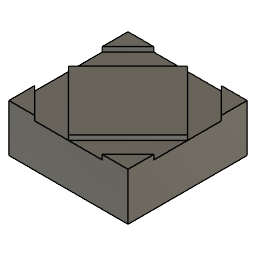
Tugas CNC Milling (Autodesk Fusion 360 design; units mm, degrees)
part number: 2026-05-23-22-12-12-129
Autodesk Fusion 360 part; units mm, degrees
sketch "Sketch1" plane through (0, 0, 0) normal (0, 0, 1) x (1, 0, 0)
  line L0 (0, 0) -> (50, 0)
  line L1 (50, 0) -> (50, 50)
  line L2 (50, 50) -> (0, 50)
  line L3 (0, 50) -> (0, 0)
  dimension "d1" = 50
  dimension "d2" = 50
  constraint horizontal L0
  constraint vertical L1
  constraint horizontal L2
  constraint vertical L3
  constraint coincident L0.start L3.end
  measures "d1" distance of L0.end L1.end
  measures "d2" distance of L1.end L2.end
extrude "Extrude1" add sketch "Sketch1" along normal blind 20
sketch "Sketch2" plane through (0, 0, 20) normal (0, 0, 1) x (-1, 0, 0)
  line L0 (0, -50) -> (0, 0)
  line L1 (0, 0) -> (-50, 0)
  line L2 (-50, 0) -> (-50, -50)
  line L3 (-50, -50) -> (0, -50)
  line L4 (-25, 0) -> (0, -25)
  line L5 (0, -25) -> (-25, -50)
  line L6 (-25, -50) -> (-50, -25)
  line L7 (-50, -25) -> (-25, 0)
  line L8 (0, -10.8579) -> (-10.8579, 0)
  line L9 (-39.1421, 0) -> (-50, -10.8579)
  line L10 (-50, -39.1421) -> (-39.1421, -50)
  line L11 (-10.8579, -50) -> (0, -39.1421)
  line L12 (0, -10.8579) -> (0, -39.1421)
  line L13 (-10.8579, -50) -> (-39.1421, -50)
  line L14 (-50, -39.1421) -> (-50, -10.8579)
  line L15 (-39.1421, 0) -> (-10.8579, 0)
  dimension "d5" = 10
  dimension "d6" = 10
  dimension "d7" = 10
  dimension "d8" = 10
  constraint midpoint L1 L4.start
  constraint midpoint L0 L4.end
  constraint midpoint L3 L5.end
  constraint midpoint L2 L6.end
  constraint coincident L0 L8.start
  constraint coincident L1 L8.end
  constraint perpendicular L7 L8
  constraint coincident L1 L9.start
  constraint coincident L2 L9.end
  constraint perpendicular L4 L9
  constraint coincident L2 L10.start
  constraint coincident L3 L10.end
  constraint perpendicular L9 L10
  constraint coincident L3 L11.start
  constraint coincident L0 L11.end
  constraint perpendicular L10 L11
  measures "d5" distance of L6 L10
  measures "d6" distance of L7 L9
  measures "d7" distance of L4 L8
  measures "d8" distance of L5 L11
extrude "Extrude2" cut sketch "Sketch2" against normal blind 2 contours L0 L3 L5 L11 L12 L13 | L0 L1 L4 L8 L12 L15 | L2 L3 L6 L10 L13 L14 | L1 L2 L7 L9 L14 L15
sketch "Sketch3" plane through (0, 0, 0) normal (0, 0, 1) x (1, 0, 0)
